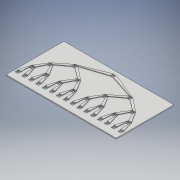
# Autodesk Inventor part: front plate
Saved by Autodesk Inventor 2018.2 (Build 222227000, 227)
## iProperties
Created: 2018-01-31
Part Number: front plate
Material: Generic
Document SubType Name: Modeling
Designer: wharr
Density: 1 g/cm^3
Appearance: Default
Author: wharr
Autodesk Inventor part; units mm, degrees
ref_plane "YZ Plane" through (0, 0, 0) normal (1, 0, 0) x (0, 1, 0)
ref_plane "XZ Plane" through (0, 0, 0) normal (0, 1, 0) x (-1, 0, 0)
ref_plane "XY Plane" through (0, 0, 0) normal (0, 0, 1) x (1, 0, 0)
sketch "Sketch1" plane through (0, 0, 0) normal (0, 0, 1) x (1, 0, 0)
  line L0 (-100, -50) -> (100, -50)
  line L1 (100, -50) -> (100, 50)
  line L2 (100, 50) -> (-100, 50)
  line L3 (-100, 50) -> (-100, -50)
  line L4 (-100, -50) -> (100, 50) construction
  line L5 (100, -50) -> (-100, 50) construction
  line L6 (-100, 30) -> (100, 30) construction
  line L7 (-100, 10) -> (100, 10) construction
  line L8 (-100, -10) -> (100, -10) construction
  line L9 (-100, -30) -> (100, -30) construction
  line L10 (-100, 40) -> (100, 40) construction
  line L11 (-2.75, 37.25) -> (2.75, 37.25)
  line L12 (2.75, 37.25) -> (2.75, 42.75)
  line L13 (2.75, 42.75) -> (-2.75, 42.75)
  line L14 (-2.75, 42.75) -> (-2.75, 37.25)
  line L15 (-2.75, 37.25) -> (2.75, 42.75) construction
  line L16 (2.75, 37.25) -> (-2.75, 42.75) construction
  line L17 (0, 50) -> (0, -50) construction
  line L18 (-50, 50) -> (-50, -50) construction
  line L19 (-100, 20) -> (100, 20) construction
  line L20 (-52.75, 17.25) -> (-47.25, 17.25)
  line L21 (-47.25, 17.25) -> (-47.25, 22.75)
  line L22 (-47.25, 22.75) -> (-52.75, 22.75)
  line L23 (-52.75, 22.75) -> (-52.75, 17.25)
  line L24 (-52.75, 17.25) -> (-47.25, 22.75) construction
  line L25 (-47.25, 17.25) -> (-52.75, 22.75) construction
  line L26 (-75, 50) -> (-75, -50) construction
  line L27 (-100, 0) -> (100, 0) construction
  line L28 (-72.25, -2.75) -> (-77.75, -2.75)
  line L29 (-77.75, -2.75) -> (-77.75, 2.75)
  line L30 (-77.75, 2.75) -> (-72.25, 2.75)
  line L31 (-72.25, 2.75) -> (-72.25, -2.75)
  line L32 (-72.25, -2.75) -> (-77.75, 2.75) construction
  line L33 (-77.75, -2.75) -> (-72.25, 2.75) construction
  line L34 (-25, 50) -> (-25, -50) construction
  line L35 (-22.25, -2.75) -> (-27.75, -2.75)
  line L36 (-27.75, -2.75) -> (-27.75, 2.75)
  line L37 (-27.75, 2.75) -> (-22.25, 2.75)
  line L38 (-22.25, 2.75) -> (-22.25, -2.75)
  line L39 (-22.25, -2.75) -> (-27.75, 2.75) construction
  line L40 (-27.75, -2.75) -> (-22.25, 2.75) construction
  line L41 (-100, -20) -> (100, -20) construction
  line L42 (-87.5, 50) -> (-87.5, -50) construction
  line L43 (-90.25, -22.75) -> (-84.75, -22.75)
  line L44 (-84.75, -22.75) -> (-84.75, -17.25)
  line L45 (-84.75, -17.25) -> (-90.25, -17.25)
  line L46 (-90.25, -17.25) -> (-90.25, -22.75)
  line L47 (-90.25, -22.75) -> (-84.75, -17.25) construction
  line L48 (-84.75, -22.75) -> (-90.25, -17.25) construction
  line L49 (-62.5, 50) -> (-62.5, -50) construction
  line L50 (-65.25, -22.75) -> (-59.75, -22.75)
  line L51 (-59.75, -22.75) -> (-59.75, -17.25)
  line L52 (-59.75, -17.25) -> (-65.25, -17.25)
  line L53 (-65.25, -17.25) -> (-65.25, -22.75)
  line L54 (-65.25, -22.75) -> (-59.75, -17.25) construction
  line L55 (-59.75, -22.75) -> (-65.25, -17.25) construction
  line L56 (-37.5, 50) -> (-37.5, -50) construction
  line L57 (-40.25, -22.75) -> (-34.75, -22.75)
  line L58 (-34.75, -22.75) -> (-34.75, -17.25)
  line L59 (-34.75, -17.25) -> (-40.25, -17.25)
  line L60 (-40.25, -17.25) -> (-40.25, -22.75)
  line L61 (-40.25, -22.75) -> (-34.75, -17.25) construction
  line L62 (-34.75, -22.75) -> (-40.25, -17.25) construction
  line L63 (-12.5, 50) -> (-12.5, -50) construction
  line L64 (-9.75, -22.75) -> (-15.25, -22.75)
  line L65 (-15.25, -22.75) -> (-15.25, -17.25)
  line L66 (-15.25, -17.25) -> (-9.75, -17.25)
  line L67 (-9.75, -17.25) -> (-9.75, -22.75)
  line L68 (-9.75, -22.75) -> (-15.25, -17.25) construction
  line L69 (-15.25, -22.75) -> (-9.75, -17.25) construction
  line L70 (-100, -40) -> (100, -40) construction
  line L71 (-93.75, -30) -> (-93.75, -50) construction
  line L72 (-81.25, -30) -> (-81.25, -50) construction
  line L73 (-96.5, -42.75) -> (-91, -42.75)
  line L74 (-91, -42.75) -> (-91, -37.25)
  line L75 (-91, -37.25) -> (-96.5, -37.25)
  line L76 (-96.5, -37.25) -> (-96.5, -42.75)
  line L77 (-96.5, -42.75) -> (-91, -37.25) construction
  line L78 (-91, -42.75) -> (-96.5, -37.25) construction
  line L79 (-68.75, -30) -> (-68.75, -50) construction
  line L80 (-56.25, -30) -> (-56.25, -50) construction
  line L81 (-43.75, -30) -> (-43.75, -50) construction
  line L82 (-31.25, -30) -> (-31.25, -50) construction
  line L83 (-18.75, -30) -> (-18.75, -50) construction
  line L84 (-6.25, -30) -> (-6.25, -50) construction
  line L85 (-84, -42.75) -> (-78.5, -42.75)
  line L86 (-78.5, -42.75) -> (-78.5, -37.25)
  line L87 (-78.5, -37.25) -> (-84, -37.25)
  line L88 (-84, -37.25) -> (-84, -42.75)
  line L89 (-84, -42.75) -> (-78.5, -37.25) construction
  line L90 (-78.5, -42.75) -> (-84, -37.25) construction
  line L91 (-71.5, -42.75) -> (-66, -42.75)
  line L92 (-66, -42.75) -> (-66, -37.25)
  line L93 (-66, -37.25) -> (-71.5, -37.25)
  line L94 (-71.5, -37.25) -> (-71.5, -42.75)
  line L95 (-71.5, -42.75) -> (-66, -37.25) construction
  line L96 (-66, -42.75) -> (-71.5, -37.25) construction
  line L97 (-59, -42.75) -> (-53.5, -42.75)
  line L98 (-53.5, -42.75) -> (-53.5, -37.25)
  line L99 (-53.5, -37.25) -> (-59, -37.25)
  line L100 (-59, -37.25) -> (-59, -42.75)
  line L101 (-59, -42.75) -> (-53.5, -37.25) construction
  line L102 (-53.5, -42.75) -> (-59, -37.25) construction
  line L103 (-46.5, -42.75) -> (-41, -42.75)
  line L104 (-41, -42.75) -> (-41, -37.25)
  line L105 (-41, -37.25) -> (-46.5, -37.25)
  line L106 (-46.5, -37.25) -> (-46.5, -42.75)
  line L107 (-46.5, -42.75) -> (-41, -37.25) construction
  line L108 (-41, -42.75) -> (-46.5, -37.25) construction
  line L109 (-34, -42.75) -> (-28.5, -42.75)
  line L110 (-28.5, -42.75) -> (-28.5, -37.25)
  line L111 (-28.5, -37.25) -> (-34, -37.25)
  line L112 (-34, -37.25) -> (-34, -42.75)
  line L113 (-34, -42.75) -> (-28.5, -37.25) construction
  line L114 (-28.5, -42.75) -> (-34, -37.25) construction
  line L115 (-21.5, -42.75) -> (-16, -42.75)
  line L116 (-16, -42.75) -> (-16, -37.25)
  line L117 (-16, -37.25) -> (-21.5, -37.25)
  line L118 (-21.5, -37.25) -> (-21.5, -42.75)
  line L119 (-21.5, -42.75) -> (-16, -37.25) construction
  line L120 (-16, -42.75) -> (-21.5, -37.25) construction
  line L121 (-9, -42.75) -> (-3.5, -42.75)
  line L122 (-3.5, -42.75) -> (-3.5, -37.25)
  line L123 (-3.5, -37.25) -> (-9, -37.25)
  line L124 (-9, -37.25) -> (-9, -42.75)
  line L125 (-9, -42.75) -> (-3.5, -37.25) construction
  line L126 (-3.5, -42.75) -> (-9, -37.25) construction
  line L127 (52.75, 17.25) -> (47.25, 17.25)
  line L128 (47.25, 17.25) -> (47.25, 22.75)
  line L129 (47.25, 22.75) -> (52.75, 22.75)
  line L130 (52.75, 22.75) -> (52.75, 17.25)
  line L131 (72.25, -2.75) -> (77.75, -2.75)
  line L132 (77.75, -2.75) -> (77.75, 2.75)
  line L133 (77.75, 2.75) -> (72.25, 2.75)
  line L134 (72.25, 2.75) -> (72.25, -2.75)
  line L135 (22.25, -2.75) -> (27.75, -2.75)
  line L136 (27.75, -2.75) -> (27.75, 2.75)
  line L137 (27.75, 2.75) -> (22.25, 2.75)
  line L138 (22.25, 2.75) -> (22.25, -2.75)
  line L139 (90.25, -22.75) -> (84.75, -22.75)
  line L140 (84.75, -22.75) -> (84.75, -17.25)
  line L141 (84.75, -17.25) -> (90.25, -17.25)
  line L142 (90.25, -17.25) -> (90.25, -22.75)
  line L143 (65.25, -22.75) -> (59.75, -22.75)
  line L144 (59.75, -22.75) -> (59.75, -17.25)
  line L145 (59.75, -17.25) -> (65.25, -17.25)
  line L146 (65.25, -17.25) -> (65.25, -22.75)
  line L147 (40.25, -22.75) -> (34.75, -22.75)
  line L148 (34.75, -22.75) -> (34.75, -17.25)
  line L149 (34.75, -17.25) -> (40.25, -17.25)
  line L150 (40.25, -17.25) -> (40.25, -22.75)
  line L151 (9.75, -22.75) -> (15.25, -22.75)
  line L152 (15.25, -22.75) -> (15.25, -17.25)
  line L153 (15.25, -17.25) -> (9.75, -17.25)
  line L154 (9.75, -17.25) -> (9.75, -22.75)
  line L155 (96.5, -42.75) -> (91, -42.75)
  line L156 (91, -42.75) -> (91, -37.25)
  line L157 (91, -37.25) -> (96.5, -37.25)
  line L158 (96.5, -37.25) -> (96.5, -42.75)
  line L159 (84, -42.75) -> (78.5, -42.75)
  line L160 (78.5, -42.75) -> (78.5, -37.25)
  line L161 (78.5, -37.25) -> (84, -37.25)
  line L162 (84, -37.25) -> (84, -42.75)
  line L163 (71.5, -42.75) -> (66, -42.75)
  line L164 (66, -42.75) -> (66, -37.25)
  line L165 (66, -37.25) -> (71.5, -37.25)
  line L166 (71.5, -37.25) -> (71.5, -42.75)
  line L167 (59, -42.75) -> (53.5, -42.75)
  line L168 (53.5, -42.75) -> (53.5, -37.25)
  line L169 (53.5, -37.25) -> (59, -37.25)
  line L170 (59, -37.25) -> (59, -42.75)
  line L171 (46.5, -42.75) -> (41, -42.75)
  line L172 (41, -42.75) -> (41, -37.25)
  line L173 (41, -37.25) -> (46.5, -37.25)
  line L174 (46.5, -37.25) -> (46.5, -42.75)
  line L175 (34, -42.75) -> (28.5, -42.75)
  line L176 (28.5, -42.75) -> (28.5, -37.25)
  line L177 (28.5, -37.25) -> (34, -37.25)
  line L178 (34, -37.25) -> (34, -42.75)
  line L179 (21.5, -42.75) -> (16, -42.75)
  line L180 (16, -42.75) -> (16, -37.25)
  line L181 (16, -37.25) -> (21.5, -37.25)
  line L182 (21.5, -37.25) -> (21.5, -42.75)
  line L183 (9, -42.75) -> (3.5, -42.75)
  line L184 (3.5, -42.75) -> (3.5, -37.25)
  line L185 (3.5, -37.25) -> (9, -37.25)
  line L186 (9, -37.25) -> (9, -42.75)
  point P0 (0, 0)
  point P1 (0, 40)
  point P2 (-50, 20)
  point P3 (-75, 0)
  point P4 (-25, 0)
  point P5 (-87.5, -20)
  point P6 (-62.5, -20)
  point P7 (-37.5, -20)
  point P8 (-12.5, -20)
  point P9 (-93.75, -40)
  point P10 (-81.25, -40)
  point P11 (-68.75, -40)
  point P12 (-56.25, -40)
  point P13 (-43.75, -40)
  point P14 (-31.25, -40)
  point P15 (-18.75, -40)
  point P16 (-6.25, -40)
  dimension "d0" = 100
  dimension "d1" = 200
  dimension "d2" = 20
  dimension "d3" = 20
  dimension "d4" = 20
  dimension "d5" = 20
  dimension "d6" = 10
  dimension "d7" = 5.5
  dimension "d8" = 5.5
  dimension "d9" = 50
  dimension "d10" = 10
  dimension "d11" = 5.5
  dimension "d12" = 5.5
  dimension "d13" = 25
  dimension "d14" = 5.5
  dimension "d15" = 5.5
  dimension "d16" = 75
  dimension "d17" = 5.5
  dimension "d18" = 5.5
  dimension "d19" = 10
  dimension "d20" = 12.5
  dimension "d21" = 5.5
  dimension "d22" = 5.5
  dimension "d23" = 37.5
  dimension "d24" = 5.5
  dimension "d25" = 5.5
  dimension "d26" = 62.5
  dimension "d27" = 5.5
  dimension "d28" = 5.5
  dimension "d29" = 87.5
  dimension "d30" = 5.5
  dimension "d31" = 5.5
  dimension "d32" = 10
  dimension "d33" = 6.25
  dimension "d34" = 12.5
  dimension "d35" = 5.5
  dimension "d36" = 5.5
  dimension "d37" = 12.5
  dimension "d38" = 12.5
  dimension "d39" = 12.5
  dimension "d40" = 12.5
  dimension "d41" = 12.5
  dimension "d42" = 12.5
  dimension "d43" = 5.5
  dimension "d44" = 5.5
  dimension "d45" = 5.5
  dimension "d46" = 5.5
  dimension "d47" = 5.5
  dimension "d48" = 5.5
  dimension "d49" = 5.5
  dimension "d50" = 5.5
  dimension "d51" = 5.5
  dimension "d52" = 5.5
  dimension "d53" = 5.5
  dimension "d54" = 5.5
  dimension "d55" = 5.5
  dimension "d56" = 5.5
  constraints: 364 end point, 60 symmetric about line, 45 midpoint, 32 parallel, 23 horizontal, 16 perpendicular, 15 vertical, 11 point on line, 65 other
  measures "d0" distance of L5.start L4.end
  measures "d1" distance of L4.end L5.end
  measures "d3" distance between parallel lines of L7 L6
  measures "d4" distance between parallel lines of L8 L7
  measures "d7" distance of L13.end L12.end
  measures "d8" distance of L12.end L11.end
  measures "d9" distance of the line from the sketch origin of L18
  measures "d10" distance between parallel lines of L6 L19
  measures "d11" distance of L22.end L21.end
  measures "d12" distance of L21.end L20.end
  measures "d14" distance of L29.end L30.end
  measures "d15" distance of L28.end L29.end
  measures "d17" distance of L36.end L37.end
  measures "d18" distance of L35.end L36.end
  measures "d19" distance between parallel lines of L8 L41
  measures "d21" distance of L45.end L44.end
  measures "d22" distance of L44.end L43.end
  measures "d24" distance of L52.end L51.end
  measures "d25" distance of L51.end L50.end
  measures "d27" distance of L59.end L58.end
  measures "d28" distance of L58.end L57.end
  measures "d30" distance of L65.end L66.end
  measures "d31" distance of L64.end L65.end
  measures "d34" distance between parallel lines of L72 L71
  measures "d35" distance of L75.end L74.end
  measures "d36" distance of L74.end L73.end
  measures "d37" distance between parallel lines of L79 L72
  measures "d38" distance between parallel lines of L80 L79
  measures "d39" distance between parallel lines of L81 L80
  measures "d40" distance between parallel lines of L82 L81
  measures "d41" distance between parallel lines of L83 L82
  measures "d42" distance between parallel lines of L84 L83
  measures "d43" distance of L87.end L86.end
  measures "d44" distance of L86.end L85.end
  measures "d45" distance of L93.end L92.end
  measures "d46" distance of L92.end L91.end
  measures "d47" distance of L99.end L98.end
  measures "d48" distance of L98.end L97.end
  measures "d49" distance of L105.end L104.end
  measures "d50" distance of L104.end L103.end
  measures "d51" distance of L111.end L110.end
  measures "d52" distance of L110.end L109.end
  measures "d53" distance of L117.end L116.end
  measures "d54" distance of L116.end L115.end
  measures "d55" distance of L123.end L122.end
  measures "d56" distance of L122.end L121.end
extrude "Extrusion1" add sketch "Sketch1" along normal blind 2
sketch "Sketch2" plane through (-100, -50, 0) normal (0, -1, 0) x (1, 0, 0)
  line L0 (0, 2) -> (200, 2) projected
  line L1 (0, 0) -> (200, 0) projected
  line L2 (200, 2) -> (0, 2)
  line L3 (0, 2) -> (0, 0)
  line L4 (0, 0) -> (200, 0)
  line L5 (200, 0) -> (200, 2)
  point P0 (100, 0)
  constraints: 8 end point, 2 parallel, 1 horizontal, 1 perpendicular
extrude "Extrusion2" add sketch "Sketch2" along normal blind 5
sketch "Sketch3" plane through (0, 0, 2) normal (0, 0, 1) x (1, 0, 0)
  line L0 (-52.75, 22.75) -> (-47.25, 22.75) projected
  line L1 (-2.75, 42.75) -> (2.75, 42.75) projected
  line L2 (-52.75, 22.75) -> (-2.75, 42.75)
  line L3 (-2.75, 37.25) -> (2.75, 37.25) projected
  line L4 (-47.25, 22.75) -> (-47.25, 17.25) projected
  line L5 (-2.75, 37.25) -> (-47.25, 22.75)
  line L6 (-77.75, 2.75) -> (-72.25, 2.75) projected
  line L7 (-52.75, 22.75) -> (-77.75, 2.75)
  line L8 (-47.25, 17.25) -> (-52.75, 17.25) projected
  line L9 (-52.75, 17.25) -> (-72.25, 2.75)
  line L10 (-22.25, 2.75) -> (-22.25, -2.75) projected
  line L11 (-47.25, 22.75) -> (-22.25, 2.75)
  line L12 (-27.75, 2.75) -> (-22.25, 2.75) projected
  line L13 (-47.25, 17.25) -> (-27.75, 2.75)
  line L14 (-77.75, -2.75) -> (-77.75, 2.75) projected
  line L15 (-90.25, -17.25) -> (-84.75, -17.25) projected
  line L16 (-77.75, 2.75) -> (-90.25, -17.25)
  line L17 (-72.25, -2.75) -> (-77.75, -2.75) projected
  line L18 (-84.75, -17.25) -> (-84.75, -22.75) projected
  line L19 (-77.75, -2.75) -> (-84.75, -17.25)
  line L20 (-59.75, -22.75) -> (-65.25, -22.75) projected
  line L21 (-72.25, 2.75) -> (-72.25, -2.75) projected
  line L22 (-59.75, -17.25) -> (-59.75, -22.75) projected
  line L23 (-72.25, 2.75) -> (-59.75, -17.25)
  line L24 (-65.25, -22.75) -> (-65.25, -17.25) projected
  line L25 (-72.25, -2.75) -> (-65.25, -17.25)
  line L26 (-96.5, -42.75) -> (-96.5, -37.25) projected
  line L27 (-90.25, -17.25) -> (-96.5, -37.25)
  line L28 (-84.75, -22.75) -> (-90.25, -22.75) projected
  line L29 (-91, -37.25) -> (-91, -42.75) projected
  line L30 (-90.25, -22.75) -> (-91, -37.25)
  line L31 (-84, -37.25) -> (-78.5, -37.25) projected
  line L32 (-84.75, -22.75) -> (-84, -37.25)
  line L33 (-78.5, -37.25) -> (-78.5, -42.75) projected
  line L34 (-84.75, -17.25) -> (-78.5, -37.25)
  line L35 (-71.5, -37.25) -> (-66, -37.25) projected
  line L36 (-65.25, -17.25) -> (-71.5, -37.25)
  line L37 (-65.25, -22.75) -> (-66, -37.25)
  line L38 (-53.5, -37.25) -> (-53.5, -42.75) projected
  line L39 (-59.75, -17.25) -> (-53.5, -37.25)
  line L40 (-59, -37.25) -> (-53.5, -37.25) projected
  line L41 (-59.75, -22.75) -> (-59, -37.25)
  line L42 (-40.25, -17.25) -> (-34.75, -17.25) projected
  line L43 (-40.25, -17.25) -> (-27.75, 2.75)
  line L44 (-22.25, -2.75) -> (-27.75, -2.75) projected
  line L45 (-27.75, -2.75) -> (-34.75, -17.25)
  line L46 (-46.5, -37.25) -> (-41, -37.25) projected
  line L47 (-40.25, -17.25) -> (-46.5, -37.25)
  line L48 (-34.75, -22.75) -> (-40.25, -22.75) projected
  line L49 (-40.25, -22.75) -> (-41, -37.25)
  line L50 (-28.5, -37.25) -> (-28.5, -42.75) projected
  line L51 (-34.75, -17.25) -> (-28.5, -37.25)
  line L52 (-34, -37.25) -> (-28.5, -37.25) projected
  line L53 (-34, -37.25) -> (-34.75, -22.75)
  line L54 (-15.25, -17.25) -> (-9.75, -17.25) projected
  line L55 (-22.25, -2.75) -> (-15.25, -17.25)
  line L56 (-9.75, -17.25) -> (-9.75, -22.75) projected
  line L57 (-22.25, 2.75) -> (-9.75, -17.25)
  line L58 (-15.25, -22.75) -> (-15.25, -17.25) projected
  line L59 (-21.5, -37.25) -> (-16, -37.25) projected
  line L60 (-15.25, -17.25) -> (-21.5, -37.25)
  line L61 (-16, -37.25) -> (-16, -42.75) projected
  line L62 (-15.25, -22.75) -> (-16, -37.25)
  line L63 (-3.5, -37.25) -> (-9, -37.25) projected
  line L64 (-9.75, -17.25) -> (-3.5, -37.25)
  line L65 (-9, -37.25) -> (-9, -42.75) projected
  line L66 (-9, -37.25) -> (-9.75, -22.75)
  line L67 (0, 50.0537) -> (0, -55) construction
  line L68 (100, -55) -> (-100, -55) construction
  line L69 (52.75, 22.75) -> (2.75, 42.75)
  line L70 (2.75, 37.25) -> (47.25, 22.75)
  line L71 (52.75, 22.75) -> (77.75, 2.75)
  line L72 (52.75, 17.25) -> (72.25, 2.75)
  line L73 (47.25, 22.75) -> (22.25, 2.75)
  line L74 (47.25, 17.25) -> (27.75, 2.75)
  line L75 (77.75, 2.75) -> (90.25, -17.25)
  line L76 (77.75, -2.75) -> (84.75, -17.25)
  line L77 (72.25, 2.75) -> (59.75, -17.25)
  line L78 (72.25, -2.75) -> (65.25, -17.25)
  line L79 (90.25, -17.25) -> (96.5, -37.25)
  line L80 (90.25, -22.75) -> (91, -37.25)
  line L81 (84.75, -22.75) -> (84, -37.25)
  line L82 (84.75, -17.25) -> (78.5, -37.25)
  line L83 (65.25, -17.25) -> (71.5, -37.25)
  line L84 (65.25, -22.75) -> (66, -37.25)
  line L85 (59.75, -17.25) -> (53.5, -37.25)
  line L86 (59.75, -22.75) -> (59, -37.25)
  line L87 (40.25, -17.25) -> (27.75, 2.75)
  line L88 (27.75, -2.75) -> (34.75, -17.25)
  line L89 (40.25, -17.25) -> (46.5, -37.25)
  line L90 (40.25, -22.75) -> (41, -37.25)
  line L91 (34.75, -17.25) -> (28.5, -37.25)
  line L92 (34, -37.25) -> (34.75, -22.75)
  line L93 (22.25, -2.75) -> (15.25, -17.25)
  line L94 (22.25, 2.75) -> (9.75, -17.25)
  line L95 (15.25, -17.25) -> (21.5, -37.25)
  line L96 (15.25, -22.75) -> (16, -37.25)
  line L97 (9.75, -17.25) -> (3.5, -37.25)
  line L98 (9, -37.25) -> (9.75, -22.75)
  line L99 (-2.75, 37.25) -> (-2.75, 42.75) projected
  line L100 (-2.75, 42.75) -> (-2.75, 37.25)
  line L101 (-52.75, 22.75) -> (-47.25, 22.75)
  line L102 (-52.75, 17.25) -> (-52.75, 22.75) projected
  line L103 (-52.75, 22.75) -> (-52.75, 17.25)
  line L104 (-47.25, 22.75) -> (-47.25, 17.25)
  line L105 (-77.75, 2.75) -> (-72.25, 2.75)
  line L106 (-77.75, 2.75) -> (-77.75, -2.75)
  line L107 (-72.25, 2.75) -> (-72.25, -2.75)
  line L108 (-27.75, 2.75) -> (-22.25, 2.75)
  line L109 (-22.25, 2.75) -> (-22.25, -2.75)
  line L110 (-27.75, 2.75) -> (-27.75, -2.75)
  line L111 (-90.25, -17.25) -> (-84.75, -17.25)
  line L112 (-84.75, -22.75) -> (-84.75, -17.25)
  line L113 (-90.25, -22.75) -> (-90.25, -17.25) projected
  line L114 (-90.25, -22.75) -> (-90.25, -17.25)
  line L115 (-65.25, -17.25) -> (-59.75, -17.25) projected
  line L116 (-65.25, -17.25) -> (-59.75, -17.25)
  line L117 (-59.75, -17.25) -> (-59.75, -22.75)
  line L118 (-65.25, -22.75) -> (-65.25, -17.25)
  line L119 (-40.25, -22.75) -> (-40.25, -17.25) projected
  line L120 (-40.25, -22.75) -> (-40.25, -17.25)
  line L121 (-40.25, -17.25) -> (-34.75, -17.25)
  line L122 (-34.75, -17.25) -> (-34.75, -22.75) projected
  line L123 (-34.75, -17.25) -> (-34.75, -22.75)
  line L124 (-15.25, -22.75) -> (-15.25, -17.25)
  line L125 (-15.25, -17.25) -> (-9.75, -17.25)
  line L126 (-9.75, -17.25) -> (-9.75, -22.75)
  line L127 (-96.5, -37.25) -> (-91, -37.25) projected
  line L128 (-96.5, -37.25) -> (-91, -37.25)
  line L129 (-84, -37.25) -> (-78.5, -37.25)
  line L130 (-71.5, -37.25) -> (-66, -37.25)
  line L131 (-59, -37.25) -> (-53.5, -37.25)
  line L132 (-46.5, -37.25) -> (-41, -37.25)
  line L133 (-34, -37.25) -> (-28.5, -37.25)
  line L134 (-21.5, -37.25) -> (-16, -37.25)
  line L135 (-9, -37.25) -> (-3.5, -37.25)
  line L136 (52.75, 22.75) -> (47.25, 22.75)
  line L137 (47.25, 22.75) -> (47.25, 17.25)
  line L138 (77.75, 2.75) -> (72.25, 2.75)
  line L139 (22.25, 2.75) -> (22.25, -2.75)
  line L140 (27.75, 2.75) -> (22.25, 2.75)
  line L141 (77.75, -2.75) -> (77.75, 2.75)
  line L142 (90.25, -17.25) -> (84.75, -17.25)
  line L143 (84.75, -17.25) -> (84.75, -22.75)
  line L144 (72.25, 2.75) -> (72.25, -2.75)
  line L145 (59.75, -17.25) -> (59.75, -22.75)
  line L146 (65.25, -22.75) -> (65.25, -17.25)
  line L147 (84, -37.25) -> (78.5, -37.25)
  line L148 (71.5, -37.25) -> (66, -37.25)
  line L149 (59, -37.25) -> (53.5, -37.25)
  line L150 (40.25, -17.25) -> (34.75, -17.25)
  line L151 (46.5, -37.25) -> (41, -37.25)
  line L152 (34, -37.25) -> (28.5, -37.25)
  line L153 (15.25, -17.25) -> (9.75, -17.25)
  line L154 (9.75, -17.25) -> (9.75, -22.75)
  line L155 (15.25, -22.75) -> (15.25, -17.25)
  line L156 (21.5, -37.25) -> (16, -37.25)
  line L157 (3.5, -37.25) -> (9, -37.25)
  line L158 (2.75, 37.25) -> (2.75, 42.75)
  line L159 (52.75, 17.25) -> (52.75, 22.75)
  line L160 (27.75, 2.75) -> (27.75, -2.75)
  line L161 (90.25, -22.75) -> (90.25, -17.25)
  line L162 (65.25, -17.25) -> (59.75, -17.25)
  line L163 (40.25, -22.75) -> (40.25, -17.25)
  line L164 (34.75, -17.25) -> (34.75, -22.75)
  line L165 (96.5, -37.25) -> (91, -37.25)
  point P0 (0, 0)
  constraints: 242 end point, 44 symmetric about line, 24 equal length, 5 perpendicular, 1 midpoint
extrude "Extrusion3" add sketch "Sketch3" along normal blind 1 contours L2 L99 L5 L0 | L79 L165 L80 L161 | L143 L81 L147 L82 | L75 L142 L76 L141 | L83 L148 L84 L146 | L145 L86 L149 L85 | L144 L78 L162 L77 | L71 L138 L72 L159 | L89 L151 L90 L163 | L164 L92 L152 L91 | L87 L150 L88 L160 | L95 L156 L96 L155 | L154 L98 L157 L97 | L139 L93 L153 L94 | L137 L74 L140 L73 | L64 L63 L66 L56 | L58 L62 L59 L60 | L102 L9 L6 L7 | L11 L12 L13 L4 | L14 L19 L15 L16 | L57 L54 L55 L10 | L69 L136 L70 L158 | L23 L115 L25 L21 | L113 L30 L127 L27 | L110 L45 L42 L43 | L39 L40 L41 L22 | L34 L31 L32 L18 | L119 L49 L46 L47 | L24 L37 L35 L36 | L51 L52 L53 L122
body "Solid1"
